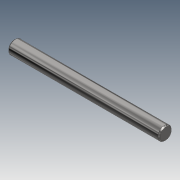
# Autodesk Inventor part: Вал промежуточный
Saved by Autodesk Inventor 2017 (Build 210142000, 142)
## iProperties
Created: 2018-08-24
Part Number: Вал промежуточный
Material: Сталь нержавеющая, 440C
Document SubType Name: Modeling
Designer: Shepelev
Density: 7.75 g/cm^3
Appearance: С умеренной полировкой
Author: Shepelev
Autodesk Inventor part; units mm, degrees
ref_plane "YZ Plane" through (0, 0, 0) normal (1, 0, 0) x (0, 1, 0)
ref_plane "XZ Plane" through (0, 0, 0) normal (0, 1, 0) x (-1, 0, 0)
ref_plane "XY Plane" through (0, 0, 0) normal (0, 0, 1) x (1, 0, 0)
sketch "Эскиз1" plane through (0, 0, 0) normal (1, 0, 0) x (0, 1, 0)
  circle A0 centre (0, 0) radius 0.6
  dimension "d0" = 1.2
  constraints: 1 centre point, 1 coincident
  measures "d0" diameter of A0
extrude "Выдавливание1" add sketch "Эскиз1" along normal blind 13.5
chamfer "Фаска1" distance 0.1 angle 45 2 edges at (0, -0.6, 0) (13.5, -0.6, 0)
